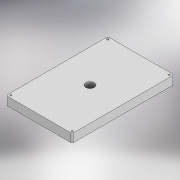
# Autodesk Inventor part: Chasis Tapa Raspberry Pi
Saved by Autodesk Inventor 2021.4 (Build 254397000, 397)
## iProperties
Created: 2022-12-12
Part Number: Chasis Tapa Raspberry Pi
Material: Genérico
Document SubType Name: Modeling
Designer: crist
Density: 1 g/cm^3
Appearance: Valor por defecto
Mass: 18.6943 g
Surface Area: 195.171 cm^2
Volume: 18.6943 cm^3
Author: crist
Autodesk Inventor part; units mm, degrees
ref_plane "YZ Plane" through (0, 0, 0) normal (1, 0, 0) x (0, 1, 0)
ref_plane "XZ Plane" through (0, 0, 0) normal (0, 1, 0) x (-1, 0, 0)
ref_plane "XY Plane" through (0, 0, 0) normal (0, 0, 1) x (1, 0, 0)
sketch "Boceto1" plane through (0, 0, 0) normal (0, 1, 0) x (-1, 0, 0)
  line L0 (0, 0) -> (78, 0)
  line L1 (78, 0) -> (78, -120)
  line L2 (78, -120) -> (0, -120)
  line L3 (0, -120) -> (0, 0)
  line L4 (39, -120) -> (39, -40.9916)
  line L5 (0, -60) -> (49.8561, -60)
  circle A0 centre (39, -60) radius 5
  dimension "d0" = 120
  dimension "d1" = 78
  dimension "d11" = 10
  constraints: 12 end point, 2 horizontal, 2 midpoint, 2 parallel, 2 point on line, 1 centre point, 1 perpendicular, 1 vertical
  measures "d0" distance of L0.end L1.end
  measures "d1" distance of L1.end L2.end
  measures "d11" diameter of A0
extrude "Extrusión1" add sketch "Boceto1" along normal blind 10 contours L0 L1 L2 L4 A0 L5 L3 | L5 A0 L4 L2 L3
fillet "Empalme1" radius 2 4 edges at (0, 5, 0) (-78, 5, -120) (0, 5, -120) (-78, 5, 0)
sketch "Boceto2" plane through (0, 10, 0) normal (0, 1, 0) x (1, 0, 0)
  circle A0 centre (0, 0) radius 4
  line L0 (0, 0) -> (-8.4064, 8.4064)
  arc A1 (-2, 0) -> (0, 2) centre (-2, 2) ccw
  circle A2 centre (-2.8284, 2.8284) radius 1
  line L1 (0, 60) -> (-13.3552, 60)
  line L2 (-39, 120) -> (-39, 106.5507)
  circle A3 centre (0, 120) radius 4
  line L3 (0, 120) -> (-8.4064, 111.5936)
  arc A4 (0, 118) -> (-2, 120) centre (-2, 118) ccw
  circle A5 centre (-2.8284, 117.1716) radius 1
  circle A6 centre (-78, 120) radius 4
  line L4 (-78, 120) -> (-69.5936, 111.5936)
  arc A7 (-76, 120) -> (-78, 118) centre (-76, 118) ccw
  circle A8 centre (-75.1716, 117.1716) radius 1
  circle A9 centre (-78, 0) radius 4
  line L5 (-78, 0) -> (-69.5936, 8.4064)
  arc A10 (-78, 2) -> (-76, 0) centre (-76, 2) ccw
  circle A11 centre (-75.1716, 2.8284) radius 1
  dimension "d5" = 8
  dimension "d8" = 2
  constraints: 24 symmetric about line, 12 end point, 8 centre point, 8 coincident, 8 point on circle, 4 point on line, 3 horizontal, 2 vertical, 18 other
  measures "d8" diameter of A2
extrude "Extrusión2" cut sketch "Boceto2" against normal blind 2 contours A2 L0 A0 | A0 L0 A2 | A2 L0 A0 | A0 L0 A2 | A5 L3 A3 | A3 L3 A5 | A5 L3 A3 | A3 L3 A5 | A8 L4 A6 | A6 L4 A8 | A8 L4 A6 | A6 L4 A8 | A11 L5 A9 | A9 L5 A11 | A11 L5 A9 | A9 L5 A11
equation "\"d2\" = d11"
